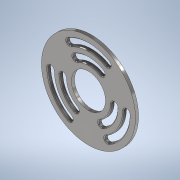
# Autodesk Inventor part: Ограничитель
Saved by Autodesk Inventor 2021 (Build 250183000, 183)
## iProperties
Created: 2020-12-19
Part Number: Ограничитель
Material: Сталь, высокопрочная, низколегированная
Document SubType Name: Modeling
Designer: Тимоха
Mass: 250.783 g
Surface Area: 205.946 cm^2
Volume: 31.9469 cm^3
Density: 7.85 g/cm^3
Appearance: Сталь — полированная
Author: Тимоха
Autodesk Inventor part; units mm, degrees
ref_plane "YZ Plane" through (0, 0, 0) normal (1, 0, 0) x (0, 1, 0)
ref_plane "XZ Plane" through (0, 0, 0) normal (0, 1, 0) x (-1, 0, 0)
ref_plane "XY Plane" through (0, 0, 0) normal (0, 0, 1) x (1, 0, 0)
sketch "Эскиз1" plane through (0, 0, 0) normal (0, 0, 1) x (1, 0, 0)
  circle A0 centre (0, 0) radius 62
  circle A1 centre (0, 0) radius 22.5
  dimension "d0" = 124
  dimension "d15" = 45
  constraints: 2 centre point, 2 coincident
  measures "d0" diameter of A0
  measures "d15" diameter of A1
extrude "Выдавливание1" add sketch "Эскиз1" along normal blind 4
sketch "Эскиз2" plane through (0, 0, 4) normal (0, 0, 1) x (1, 0, 0)
  arc A0 (17, 29.4449) -> (-17, 29.4449) centre (0, 0) ccw construction
  arc A1 (19, 32.909) -> (-19, 32.909) centre (0, 0) ccw
  arc A2 (15, 25.9808) -> (-15, 25.9808) centre (0, 0) ccw
  arc A3 (15, 25.9808) -> (19, 32.909) centre (17, 29.4449) ccw
  arc A4 (-19, 32.909) -> (-15, 25.9808) centre (-17, 29.4449) ccw
  line L0 (0, 0) -> (-17, 29.4449) construction
  line L1 (0, 0) -> (34, 0) construction
  line L2 (0, 0) -> (17, 29.4449) construction
  arc A5 (25, 43.3013) -> (-25, 43.3013) centre (0, 0) ccw construction
  arc A6 (27, 46.7654) -> (-27, 46.7654) centre (0, 0) ccw
  arc A7 (23, 39.8372) -> (-23, 39.8372) centre (0, 0) ccw
  arc A8 (23, 39.8372) -> (27, 46.7654) centre (25, 43.3013) ccw
  arc A9 (-27, 46.7654) -> (-23, 39.8372) centre (-25, 43.3013) ccw
  line L3 (0, 0) -> (-25, 43.3013) construction
  line L4 (0, 0) -> (50, 0) construction
  line L5 (0, 0) -> (25, 43.3013) construction
  arc A10 (33, 57.1577) -> (-33, 57.1577) centre (0, 0) ccw construction
  line L6 (0, 0) -> (-33, 57.1577) construction
  line L7 (0, 0) -> (66, 0) construction
  line L8 (0, 0) -> (33, 57.1577) construction
  dimension "d3" = 34
  dimension "d4" = 120
  dimension "d5" = 60
  dimension "d6" = 8
  dimension "d7" = 50
  dimension "d8" = 120
  dimension "d9" = 60
  dimension "d10" = 8
  dimension "d11" = 66
  dimension "d12" = 120
  dimension "d13" = 60
  constraints: 22 point on circle, 18 end point, 11 centre point, 8 tangent, 3 coincident, 3 equal length, 3 horizontal
  measures "d3" radius of A0
  measures "d4" angle of L1 L0
  measures "d5" angle of L2 L0
  measures "d6" diameter of A3
  measures "d7" radius of A5
  measures "d8" angle of L4 L3
  measures "d9" angle of L5 L3
  measures "d10" diameter of A8
  measures "d11" radius of A10
  measures "d12" angle of L7 L6
  measures "d13" angle of L8 L6
extrude "Выдавливание2" cut sketch "Эскиз2" against normal through all
chamfer "Фаска1" distance 1 angle 45 8 edges at (0, 54, 4) (28.4641, 41.3013, 4) (0, 46, 4) (-28.4641, 41.3013, 4) (0, 38, 4) (20.4641, 27.4449, 4) (0, 30, 4) (-20.4641, 27.4449, 4)
pattern_circular "Круговой массив1" count 3 over 360 about axis through (0, 0, 0) along (0, 0, 1) of "Выдавливание2", "Фаска1"
